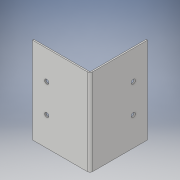
# Autodesk Inventor part: clamp
Saved by Autodesk Inventor 2019 (Build 230136000, 136)
## iProperties
Created: 2020-02-14
Part Number: clamp
Material: Generic
Document SubType Name: Modeling
Designer: Dell
Density: 1 g/cm^3
Appearance: Default
Author: Dell
Autodesk Inventor part; units mm, degrees
ref_plane "YZ Plane" through (0, 0, 0) normal (1, 0, 0) x (0, 1, 0)
ref_plane "XZ Plane" through (0, 0, 0) normal (0, 1, 0) x (-1, 0, 0)
ref_plane "XY Plane" through (0, 0, 0) normal (0, 0, 1) x (1, 0, 0)
sketch "Sketch1" plane through (0, 0, 0) normal (0, 1, 0) x (-1, 0, 0)
  line L0 (60, 0) -> (60, -1)
  line L1 (1, -60) -> (0, -60)
  line L2 (0, 0) -> (0, -40)
  line L3 (1, -1) -> (1, -40)
  line L4 (1, -40) -> (0, -40)
  line L5 (0, 0) -> (40, 0)
  line L6 (1, -1) -> (40, -1)
  line L7 (40, -1) -> (40, 0)
  dimension "d0" = 60
  dimension "d2" = 1
  dimension "d15" = 40
  dimension "d24" = 40
  constraints: 16 end point, 2 horizontal, 2 perpendicular, 2 vertical, 1 parallel
  measures "d0" distance of L2.start L1.end
  measures "d2" distance of L0.start L0.end
  measures "d15" distance of L2.start L2.end
  measures "d24" distance of L2.start L5.end
extrude "Extrusion1" add sketch "Sketch1" along normal blind 60
fillet "Fillet1" radius 2 1 edges at (0, 30, 0)
sketch "Sketch4" plane through (0, 0, -40) normal (1, 0, 0) x (0, 0, -1)
  circle A0 centre (-10, 40) radius 1.5
  circle A1 centre (-10, 20) radius 1.5
  point P0 (-40, 0)
  dimension "d17" = 3
  dimension "d18" = 3
  constraints: 2 centre point
  measures "d17" diameter of A0
  measures "d18" diameter of A1
extrude "Extrusion4" cut sketch "Sketch4" against normal blind 1
sketch "Sketch5" plane through (-40, 0, 0) normal (0, 0, 1) x (1, 0, 0)
  circle A0 centre (10, 40) radius 1.5
  circle A1 centre (10, 20) radius 1.5
  point P0 (40, 0)
  dimension "d25" = 3
  dimension "d27" = 3
  constraints: 2 centre point
  measures "d25" diameter of A0
  measures "d27" diameter of A1
extrude "Extrusion5" cut sketch "Sketch5" against normal blind 1
body "Solid1"
